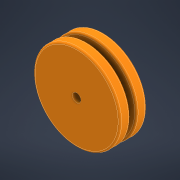
# Autodesk Inventor part: bushing_smConnection
Saved by Autodesk Inventor 2021 (Build 250183000, 183)
## iProperties
Created: 2021-06-22
Part Number: bushing_smConnection
Material: Generic
Document SubType Name: Modeling
Designer: Watchdog
Density: 1 g/cm^3
Appearance: Orange
Author: Watchdog
Autodesk Inventor part; units mm, degrees
ref_plane "YZ Plane" through (0, 0, 0) normal (1, 0, 0) x (0, 1, 0)
ref_plane "XZ Plane" through (0, 0, 0) normal (0, 1, 0) x (-1, 0, 0)
ref_plane "XY Plane" through (0, 0, 0) normal (0, 0, 1) x (1, 0, 0)
sketch "Sketch1" plane through (0, 0, 0) normal (0, 1, 0) x (-1, 0, 0)
  line L0 (50, -15.5) -> (5, -15.5)
  line L1 (5, 15.5) -> (50, 15.5)
  line L2 (50, 15.5) -> (50, 3.5)
  line L3 (50, 3.5) -> (15, 3.5)
  line L4 (15, 3.5) -> (15, -3.5)
  line L5 (15, -3.5) -> (50, -3.5)
  line L6 (50, -3.5) -> (50, -15.5)
  line L7 (0, 147.0752) -> (0, -168.5589)
  line L8 (5, 15.5) -> (5, -15.5)
  point P0 (0, 0)
  dimension "d6" = 12
  dimension "d7" = 12
  dimension "d10" = 3.5
  dimension "d11" = 7
  dimension "d15" = 5
  dimension "d16" = 15
  dimension "d17" = 50
  dimension "d18" = 50
  constraints: 18 end point, 4 perpendicular, 1 horizontal, 1 parallel, 1 point on line, 1 vertical
  measures "d6" distance between parallel lines of L0 L5
  measures "d7" distance between parallel lines of L1 L3
  measures "d10" distance from line of point (0, 0) L5
  measures "d11" distance between parallel lines of L3 L5
  measures "d15" horizontal distance of L7.end L0.end
  measures "d16" distance from line of point (0, 0) L4
  measures "d17" horizontal distance of L7.end L0.start
  measures "d18" horizontal distance of L7.end L1.end
revolve "Revolution1" add sketch "Sketch1" angle 360 about axis through (0, 0, 147.0752) along (0, 0, -1)
fillet "Fillet1" radius 2 2 edges at (15, 0, -3.5) (15, 0, 3.5)
fillet "Fillet2" radius 2 4 edges at (50, 0, 3.5) (50, 0, 15.5) (50, 0, -3.5) (50, 0, -15.5)
equation "\"d7\" = d6"
equation "\"d10\" = 0.5 * d11"
equation "\"d18\" = d17"
body "Solid1"
